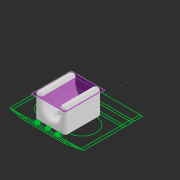
# Autodesk Inventor part: ironHolder
Saved by Autodesk Inventor 2020.3 (Build 243373010, 373A)
## iProperties
Created: 2021-04-27
Part Number: ironHolder
Material: Generic
Document SubType Name: Modeling
Designer: Melvin Strobl
Density: 1 g/cm^3
Appearance: Default
Author: Melvin Strobl
Autodesk Inventor part; units mm, degrees
ref_plane "YZ Plane" through (0, 0, 0) normal (1, 0, 0) x (0, 1, 0)
ref_plane "XZ Plane" through (0, 0, 0) normal (0, 1, 0) x (-1, 0, 0)
ref_plane "XY Plane" through (0, 0, 0) normal (0, 0, 1) x (1, 0, 0)
derived "body.ipt"
sketch "Sketch1" plane through (0, 0, 0) normal (0, 1, 0) x (-1, 0, 0)
  line L0 (0, 0) -> (53, 0)
  line L1 (53, 0) -> (53, -42.5)
  line L2 (0, -42.5) -> (0, 0)
  circle A0 centre (26.5, -32.5) radius 2.25
  line L3 (26.5, -65) -> (26.5, 0) construction
  line L4 (41.5, 0) -> (11.5, 0)
  line L5 (11.5, 0) -> (11.5, 2.5)
  line L6 (11.5, 2.5) -> (41.5, 2.5)
  line L7 (41.5, 2.5) -> (41.5, 0)
  circle A1 centre (34, -1) radius 2
  circle A2 centre (19, -1) radius 2
  line L8 (41.5, -1) -> (11.5, -1) construction
  line L9 (51, -42.5) -> (51, 0)
  line L10 (51, 0) -> (2, 0)
  line L11 (2, 0) -> (2, -42.5)
  line L12 (40.25, 1.25) -> (12.75, 1.25)
  line L13 (12.75, 1.25) -> (12.75, 1.25)
  line L14 (12.75, 1.25) -> (40.25, 1.25)
  line L15 (40.25, 1.25) -> (40.25, 1.25)
  line L16 (40.25, 1.25) -> (40.25, 0)
  line L17 (12.75, 1.25) -> (12.75, 0)
  line L18 (53, -42.5) -> (0, -42.5)
  circle A3 centre (26.5, -32.5) radius 4
  line L19 (27.75, -42.5) -> (28.25, -42.5)
  line L20 (0, -36.5) -> (53, -36.5)
  line L21 (0, -28.5) -> (53, -28.5)
  line L22 (0, -30.25) -> (53, -30.25)
  line L23 (53, -30.25) -> (53, -34.75)
  line L24 (53, -34.75) -> (0, -34.75)
  line L25 (0, -34.75) -> (0, -30.25)
  line L26 (24.4215, -36.1) -> (22.3431, -32.5)
  line L27 (22.3431, -32.5) -> (24.4215, -28.9)
  line L28 (24.4215, -28.9) -> (28.5785, -28.9)
  line L29 (28.5785, -28.9) -> (30.6569, -32.5)
  line L30 (30.6569, -32.5) -> (28.5785, -36.1)
  line L31 (28.5785, -36.1) -> (24.4215, -36.1)
  line L32 (36.5, -15.5) -> (16.5, -15.5) construction
  line L33 (36.5, -5.5) -> (16.5, -5.5)
  line L34 (16.5, -25.5) -> (36.5, -25.5)
  arc A4 (36.5, -25.5) -> (36.5, -5.5) centre (36.5, -15.5) ccw
  arc A5 (16.5, -5.5) -> (16.5, -25.5) centre (16.5, -15.5) ccw
  line L35 (41.5, 2.5) -> (53, 0)
  line L36 (11.5, 2.5) -> (0, 0)
  line L37 (12.75, 1.25) -> (2, 0)
  line L38 (40.25, 1.25) -> (51, 0)
  line L39 (19, -3) -> (34, -3)
  circle A6 centre (26.5, -1) radius 1.5
  circle A7 centre (26.5, -21.5) radius 1.6
  circle A8 centre (26.5, -9.5) radius 1.6
  point P0 (26.5, -15.5)
sketch "Sketch2" plane through (0, 0, 0) normal (0, 1, 0) x (-1, 0, 0)
  circle A0 centre (26.5, -21.5) radius 1.6 projected
  line L0 (36.5, -15.5) -> (16.5, -15.5) construction
  line L1 (26.5, -65) -> (26.5, 0) construction
  circle A1 centre (26.5, -9.5) radius 1.6 projected
  line L2 (11.5, 2.5) -> (41.5, 2.5) projected
  line L3 (53, -42.5) -> (0, -42.5) projected
  line L4 (0, -28.5) -> (53, -28.5) projected
  line L5 (33, -2.5) -> (20, -2.5)
  line L6 (20, -2.5) -> (20, -28.5)
  line L7 (20, -28.5) -> (33, -28.5)
  line L8 (33, -28.5) -> (33, -2.5)
  line L9 (33, -2.5) -> (20, -28.5) construction
  line L10 (20, -2.5) -> (33, -28.5) construction
  line L11 (37.5, -2.5) -> (15.5, -2.5)
  line L12 (15.5, -2.5) -> (15.5, -28.5)
  line L13 (15.5, -28.5) -> (37.5, -28.5)
  line L14 (37.5, -28.5) -> (37.5, -2.5)
  line L15 (37.5, -2.5) -> (15.5, -28.5) construction
  line L16 (15.5, -2.5) -> (37.5, -28.5) construction
  line L17 (26.5, -24.8486) -> (23.6, -23.1743)
  line L18 (23.6, -23.1743) -> (23.6, -19.8257)
  line L19 (23.6, -19.8257) -> (26.5, -18.1514)
  line L20 (26.5, -18.1514) -> (29.4, -19.8257)
  line L21 (29.4, -19.8257) -> (29.4, -23.1743)
  line L22 (29.4, -23.1743) -> (26.5, -24.8486)
  line L23 (26.5, -12.8486) -> (23.6, -11.1743)
  line L24 (23.6, -11.1743) -> (23.6, -7.8257)
  line L25 (23.6, -7.8257) -> (26.5, -6.1514)
  line L26 (26.5, -6.1514) -> (29.4, -7.8257)
  line L27 (29.4, -7.8257) -> (29.4, -11.1743)
  line L28 (29.4, -11.1743) -> (26.5, -12.8486)
  point P0 (0, 0)
  point P1 (26.5, -15.5)
  dimension "d1" = 13
  dimension "d2" = 22
  dimension "d3" = 5.8
  dimension "d4" = 5.8
  constraints: 48 end point, 4 midpoint, 4 parallel, 4 point on line, 2 coincident, 2 horizontal, 2 perpendicular, 26 other
  measures "d1" distance of L7.end L6.end
  measures "d2" distance of L13.end L12.end
  measures "d3" distance between parallel lines of L24 L27
  measures "d4" distance between parallel lines of L18 L21
extrude "Extrusion1" add sketch "Sketch2" along normal blind 4 contours L12 L11 L6 L4 | L6 L5 L8 L4 | L8 L11 L14 L4 | L17 L18 L19 L20 L21 L22 | L23 L24 L25 L26 L27 L28
extrude "Extrusion2" add sketch "Sketch2" along normal blind 15 contours L12 L11 L6 L4 | L8 L11 L14 L4
sketch "Sketch3" plane through (-37.5, 0, -2.5) normal (0, 0, 1) x (1, 0, 0)
  line L0 (4.5, 4) -> (4.5, 15) projected
  line L1 (17.5, 4) -> (17.5, 15) projected
  arc A0 (4.5, 10) -> (17.5, 10) centre (11, 10.5208) ccw
  line L2 (4.5, 4) -> (17.5, 4) projected
  line L3 (4.5, 4) -> (4.5, 15) projected
  arc A1 (4.5, 14.2891) -> (0, 15) centre (2.2996, 14.9587) ccw
  line L4 (17.5, 15) -> (22, 15) projected
  line L5 (17.5, 4) -> (17.5, 15) projected
  arc A2 (22, 15) -> (17.5, 14.2891) centre (19.7004, 14.9587) ccw
  line L6 (4.5, 4) -> (17.5, 4) projected
  line L7 (4.5, 4) -> (4.5, 15) projected
  line L8 (0, 15) -> (4.5, 15) projected
  line L9 (0, 0) -> (0, 15) projected
  line L10 (0, 0) -> (22, 0) projected
  line L11 (22, 0) -> (22, 15) projected
  line L12 (17.5, 15) -> (22, 15) projected
  line L13 (17.5, 4) -> (17.5, 15) projected
  point P0 (37.5, 0)
  point P1 (11, 4)
  point P2 (0, 15)
  point P3 (4.5, 14.2891)
  dimension "d9" = 6
  dimension "d10" = 6
  dimension "d13" = 2.3
  dimension "d14" = 2.3
  constraints: 6 point on circle, 4 point on line, 3 centre point, 1 tangent
  measures "d9" distance of L1.start A0.end
  measures "d10" distance of L0.start A0.start
  measures "d13" radius of A1
  measures "d14" radius of A2
extrude "Extrusion3" add sketch "Sketch3" against normal blind 26 contours L0 A0 L2 | A0 L1 L2 | L0 L8 A1 | A2 L4 L1
fillet "Fillet1" radius 2 4 edges at (-33, 14.2891, -15.5) (-20, 14.2891, -15.5) (-33, 10, -15.5) (-20, 10, -15.5)
fillet "Fillet2" radius 2 2 edges at (-37.5, 15, -15.5) (-15.5, 15, -15.5)
fillet "Fillet3" radius 2 24 edges at (-37.4994, 15.0233, -2.5) (-37.5, 7.4868, -2.5) (-32.9884, 14.2537, -2.5) (-33, 12.0192, -2.5) (-22.077, 5.7293, -2.5) (-30.923, 5.7293, -2.5) (-20.0116, 14.2537, -2.5) (-20, 12.0192, -2.5) (-18.1039, 17.2385, -2.5) (-15.5006, 15.0233, -2.5) (-15.5, 7.4868, -2.5) (-34.8961, 17.2385, -2.5) (-32.9884, 14.2537, -28.5) (-33, 12.0192, -28.5) (-22.077, 5.7293, -28.5) (-30.923, 5.7293, -28.5) (-20.0116, 14.2537, -28.5) (-20, 12.0192, -28.5) (-18.1039, 17.2385, -28.5) (-15.5006, 15.0233, -28.5) (-15.5, 7.4868, -28.5) (-37.4994, 15.0233, -28.5) (-37.5, 7.4868, -28.5) (-34.8961, 17.2385, -28.5)
ref_plane "Work Plane1" through (0, 15.25, 0) normal (0, -1, 0) x (1, 0, 0)
extrude "Extrusion4" cut sketch "Sketch2" against normal blind 13.75 from surface at 15.25 contours A0 | A1 | L17 L18 L19 L20 L21 L22 | L23 L24 L25 L26 L27 L28
fillet "Fillet4" radius 0.4 2 edges at (-24.9, 0, -21.5) (-24.9, 0, -9.5)
fillet "Fillet5" radius 0.2 8 edges at (-15.5, 0, -15.5) (-16.0858, 0, -27.9142) (-26.5, 0, -28.5) (-36.9142, 0, -27.9142) (-37.5, 0, -15.5) (-36.9142, 0, -3.0858) (-26.5, 0, -2.5) (-16.0858, 0, -3.0858)
equation "\"d4\" = d3"
equation "\"d10\" = d9"
equation "\"d14\" = d13"
body "Solid1"
